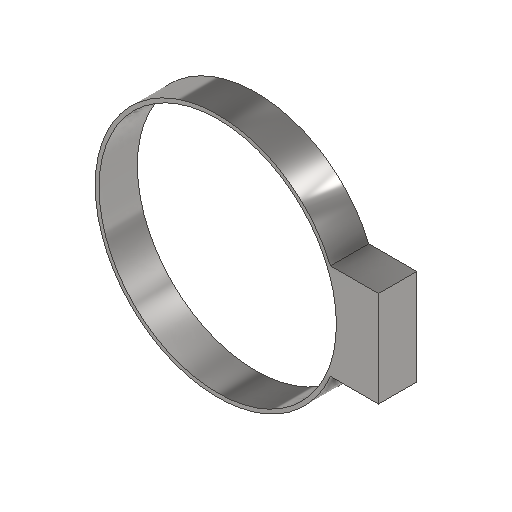
# Autodesk Inventor part: COTS_GENERIC_60mm_Hose_Clamp
Saved by Autodesk Inventor 2025 (Build 290162010, 162A)
## iProperties
Created: 2024-10-12
Part Number: COTS_GENERIC_60mm_Hose_Clamp
Material: Generic
Document SubType Name: Modeling
Designer: User
Density: 1 g/cm^3
Appearance: Steel - Polished
Author: User
Autodesk Inventor part; units mm, degrees
ref_plane "YZ Plane" through (0, 0, 0) normal (1, 0, 0) x (0, 1, 0)
ref_plane "XZ Plane" through (0, 0, 0) normal (0, 1, 0) x (-1, 0, 0)
ref_plane "XY Plane" through (0, 0, 0) normal (0, 0, 1) x (1, 0, 0)
sketch "Sketch1" plane through (0, 0, 0) normal (0, 0, 1) x (1, 0, 0)
  circle A0 centre (0, 0) radius 31
  circle A1 centre (0, 0) radius 32
  line L0 (29.4576, -12.5) -> (42, -12.5)
  line L1 (42, -12.5) -> (42, 12.5)
  line L2 (42, 12.5) -> (29.4576, 12.5)
  dimension "d0" = 62
  dimension "d1" = 1
  dimension "d2" = 25
  dimension "d3" = 10
  dimension "d4" = 12.5
  constraints: 6 end point, 2 centre point, 2 perpendicular, 2 point on circle, 1 coincident, 1 horizontal
  measures "d0" diameter of A0
  measures "d1" radial gap between concentric circles of A0 A1
  measures "d2" distance between parallel lines of L0 L2
  measures "d3" distance edge to line of A1 L1
  measures "d4" distance from line of point (0, 0) L2
extrude "Extrusion1" add sketch "Sketch1" along normal blind 10
equation "\"d4\" = 0.5 * d2"
body "Solid1"
